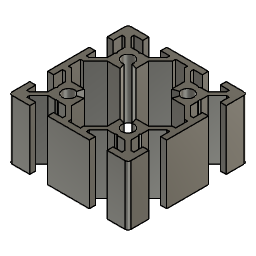
Misumi 4040 Cube (Autodesk Fusion 360 design; units mm, degrees)
Autodesk Fusion 360 part; units mm, degrees
sketch "Sketch1" plane through (0, 0, 0) normal (0, 0, 1) x (1, 0, 0)
  line L0 (14, 12.9393) -> (17.0607, 16)
  arc A0 (20, 19) -> (19, 20) centre (19, 19) ccw
  line L1 (18, 16) -> (18, 13)
  line L2 (17.0607, 4) -> (14, 7.0607)
  line L3 (-7, 20) -> (-7, 18)
  line L4 (-7, 18) -> (-4, 18)
  line L5 (-4, 18) -> (-4, 17.0607)
  line L6 (14, 9.4804) -> (13.7, 10)
  line L7 (9.4804, 14) -> (7.0607, 14)
  line L8 (14, 10.5196) -> (14, 12.9393)
  line L9 (12.9393, 14) -> (10.5196, 14)
  line L10 (7, 18) -> (7, 20)
  line L11 (20, 13) -> (20, 19)
  line L12 (14, 7.0607) -> (14, 9.4804)
  line L13 (17.0607, 16) -> (18, 16)
  line L14 (7, 20) -> (-7, 20)
  line L15 (20, 7) -> (18, 7)
  line L16 (13, 18) -> (16, 18)
  line L17 (7.0607, 14) -> (4, 17.0607)
  line L18 (4, 18) -> (7, 18)
  line L19 (18, 4) -> (17.0607, 4)
  line L20 (16, 18) -> (16, 17.0607)
  line L21 (10, 13.7) -> (9.4804, 14)
  line L22 (20, -7) -> (20, 7)
  line L23 (16, 17.0607) -> (12.9393, 14)
  line L24 (18, 7) -> (18, 4)
  line L25 (13.7, 10) -> (14, 10.5196)
  line L26 (18, 13) -> (20, 13)
  line L27 (10.5196, 14) -> (10, 13.7)
  line L28 (4, 17.0607) -> (4, 18)
  line L29 (13, 20) -> (13, 18)
  line L30 (19, 20) -> (13, 20)
  line L31 (-7, -18) -> (-7, -20)
  line L32 (7.0607, -14) -> (9.4804, -14)
  line L33 (16, -17.0607) -> (16, -18)
  line L34 (-18, 16) -> (-17.0607, 16)
  line L35 (-14, -9.4804) -> (-13.7, -10)
  line L36 (-18, 7) -> (-20, 7)
  line L37 (-18, -13) -> (-20, -13)
  line L38 (-16, 17.0607) -> (-16, 18)
  line L39 (-18, 13) -> (-18, 16)
  line L40 (-14, 12.9393) -> (-14, 10.5196)
  line L41 (-14, -7.0607) -> (-14, -9.4804)
  line L42 (-12.9393, -14) -> (-10.5196, -14)
  line L43 (-17.0607, 16) -> (-14, 12.9393)
  line L44 (-13.7, -10) -> (-14, -10.5196)
  line L45 (-16, -17.0607) -> (-12.9393, -14)
  line L46 (-14, -12.9393) -> (-17.0607, -16)
  line L47 (-16, -18) -> (-16, -17.0607)
  line L48 (-13, 18) -> (-13, 20)
  line L49 (-7.0607, -14) -> (-4, -17.0607)
  line L50 (-16, 18) -> (-13, 18)
  line L51 (-9.4804, 14) -> (-10, 13.7)
  line L52 (-10, 13.7) -> (-10.5196, 14)
  line L53 (-13, -18) -> (-16, -18)
  line L54 (-4, 17.0607) -> (-7.0607, 14)
  line L55 (-18, -16) -> (-18, -13)
  line L56 (-9.4804, -14) -> (-7.0607, -14)
  line L57 (-7, -20) -> (7, -20)
  line L58 (-20, -13) -> (-20, -19)
  line L59 (-10, -13.7) -> (-9.4804, -14)
  line L60 (-13, 20) -> (-19, 20)
  line L61 (-14, 10.5196) -> (-13.7, 10)
  line L62 (-17.0607, 4) -> (-18, 4)
  line L63 (7, -18) -> (4, -18)
  line L64 (-18, -7) -> (-18, -4)
  line L65 (-19, -20) -> (-13, -20)
  line L66 (10.5196, -14) -> (12.9393, -14)
  line L67 (7, -20) -> (7, -18)
  line L68 (-20, 7) -> (-20, -7)
  line L69 (-17.0607, -16) -> (-18, -16)
  line L70 (-14, 7.0607) -> (-17.0607, 4)
  arc A1 (-20, -19) -> (-19, -20) centre (-19, -19) ccw
  line L71 (4, -18) -> (4, -17.0607)
  line L72 (16, -18) -> (13, -18)
  line L73 (-17.0607, -4) -> (-14, -7.0607)
  line L74 (-4, -18) -> (-7, -18)
  line L75 (-14, 9.4804) -> (-14, 7.0607)
  line L76 (13, -20) -> (19, -20)
  line L77 (-7.0607, 14) -> (-9.4804, 14)
  line L78 (9.4804, -14) -> (10, -13.7)
  line L79 (18, -4) -> (18, -7)
  line L80 (-4, -17.0607) -> (-4, -18)
  line L81 (10, -13.7) -> (10.5196, -14)
  line L82 (-12.9393, 14) -> (-16, 17.0607)
  line L83 (-10.5196, -14) -> (-10, -13.7)
  line L84 (-20, 19) -> (-20, 13)
  line L85 (-10.5196, 14) -> (-12.9393, 14)
  line L86 (-13, -20) -> (-13, -18)
  line L87 (-20, 13) -> (-18, 13)
  line L88 (-20, -7) -> (-18, -7)
  line L89 (-18, -4) -> (-17.0607, -4)
  arc A2 (-19, 20) -> (-20, 19) centre (-19, 19) ccw
  line L90 (20, -19) -> (20, -13)
  line L91 (12.9393, -14) -> (16, -17.0607)
  line L92 (14, -12.9393) -> (14, -10.5196)
  line L93 (14, -10.5196) -> (13.7, -10)
  line L94 (13.7, -10) -> (14, -9.4804)
  line L95 (-14, -10.5196) -> (-14, -12.9393)
  line L96 (-18, 4) -> (-18, 7)
  line L97 (4, -17.0607) -> (7.0607, -14)
  line L98 (-13.7, 10) -> (-14, 9.4804)
  line L99 (14, -7.0607) -> (17.0607, -4)
  line L100 (18, -16) -> (17.0607, -16)
  line L101 (18, -13) -> (18, -16)
  line L102 (20, -13) -> (18, -13)
  line L103 (13, -18) -> (13, -20)
  line L104 (17.0607, -16) -> (14, -12.9393)
  arc A3 (19, -20) -> (20, -19) centre (19, -19) ccw
  line L105 (17.0607, -4) -> (18, -4)
  line L106 (18, -7) -> (20, -7)
  line L107 (14, -9.4804) -> (14, -7.0607)
  line L108 (6, 8.6667) -> (8.0078, 9.3359)
  line L109 (16.9393, -2) -> (12.9393, -6)
  arc A4 (9.3359, -8.0078) -> (8.0078, -9.3359) centre (10, -10) cw
  line L110 (-18, -2) -> (-18, 2)
  line L111 (18, -2) -> (16.9393, -2)
  line L112 (-2, 16.9393) -> (-2, 18)
  line L113 (-8.0078, 9.3359) -> (-6, 8.6667)
  line L114 (2, -16.9393) -> (2, -18)
  line L115 (12.9393, 6) -> (16.9393, 2)
  line L116 (-18, 2) -> (-16.9393, 2)
  line L117 (-9.3359, -8.0078) -> (-8.6667, -6)
  line L118 (-6, -8.6667) -> (-8.0078, -9.3359)
  line L119 (-12.9393, 6) -> (-8.6667, 6)
  line L120 (2, 18) -> (2, 16.9393)
  arc A5 (8.0078, 9.3359) -> (9.3359, 8.0078) centre (10, 10) cw
  line L121 (-6, -12.9393) -> (-6, -8.6667)
  line L122 (-16.9393, 2) -> (-12.9393, 6)
  line L123 (6, -12.9393) -> (2, -16.9393)
  line L124 (8.6667, -6) -> (9.3359, -8.0078)
  line L125 (-8.6667, -6) -> (-12.9393, -6)
  line L126 (-16.9393, -2) -> (-18, -2)
  line L127 (-2, -16.9393) -> (-6, -12.9393)
  line L128 (18, 2) -> (18, -2)
  line L129 (-2, 18) -> (2, 18)
  line L130 (-2, -18) -> (-2, -16.9393)
  line L131 (2, -18) -> (-2, -18)
  line L132 (12.9393, -6) -> (8.6667, -6)
  line L133 (-12.9393, -6) -> (-16.9393, -2)
  line L134 (6, 12.9393) -> (6, 8.6667)
  arc A6 (-8.0078, -9.3359) -> (-9.3359, -8.0078) centre (-10, -10) cw
  line L135 (2, 16.9393) -> (6, 12.9393)
  line L136 (9.3359, 8.0078) -> (8.6667, 6)
  line L137 (8.6667, 6) -> (12.9393, 6)
  line L138 (-6, 12.9393) -> (-2, 16.9393)
  line L139 (16.9393, 2) -> (18, 2)
  line L140 (8.0078, -9.3359) -> (6, -8.6667)
  line L141 (6, -8.6667) -> (6, -12.9393)
  arc A7 (-9.3359, 8.0078) -> (-8.0078, 9.3359) centre (-10, 10) cw
  line L142 (-6, 8.6667) -> (-6, 12.9393)
  line L143 (-8.6667, 6) -> (-9.3359, 8.0078)
extrude "Extrude1" add sketch "Sketch1" along normal blind 20
